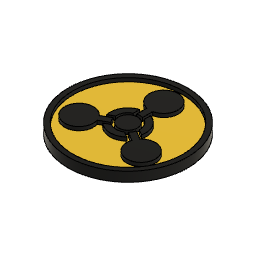
Chemical_symbol (Autodesk Fusion 360 design; units mm, degrees)
Autodesk Fusion 360 part; units mm, degrees
sketch "Sketch1" plane through (0, 0, 0) normal (0, 0, 1) x (1, 0, 0)
  circle A0 centre (0, 0) radius 25
  dimension "d1" = 50
  constraint coincident A0.centre origin
  measures "d1" diameter of A0
extrude "Extrude1" add sketch "Sketch1" along normal blind 2.5
sketch "Sketch2" plane through (0, 0, 2.5) normal (0, 0, 1) x (-1, 0, 0)
  circle A0 centre (0, 0) radius 25
  circle A1 centre (0, 0) radius 23
  circle A2 centre (0, 0) radius 21 construction
  circle A3 centre (0, 0) radius 4
  line L0 (0, 0) -> (0, -21) construction
  line L1 (0, 0) -> (-18.1865, 10.5) construction
  line L2 (18.1865, 10.5) -> (0, 0) construction
  line L3 (18.1865, 10.5) -> (0, -21) construction
  line L4 (-18.1865, 10.5) -> (0, -21) construction
  line L5 (-18.1865, 10.5) -> (18.1865, 10.5) construction
  circle A4 centre (0, 0) radius 5
  circle A5 centre (0, 0) radius 15 construction
  circle A6 centre (0, -15) radius 6
  circle A7 centre (-12.9904, 7.5) radius 6
  circle A8 centre (12.9904, 7.5) radius 6
  line L6 (8.5332, 3.4833) -> (3.9156, 0.8173)
  line L7 (7.2832, 5.6484) -> (2.6656, 2.9824)
  line L8 (8.5332, 3.4833) -> (7.2832, 5.6484) construction
  line L9 (3.9156, 0.8173) -> (2.6656, 2.9824) construction
  line L10 (-7.2832, 5.6484) -> (-2.6656, 2.9824)
  line L11 (-8.5332, 3.4833) -> (-3.9156, 0.8173)
  line L12 (-2.6656, 2.9824) -> (-3.9156, 0.8173) construction
  line L13 (-7.2832, 5.6484) -> (-8.5332, 3.4833) construction
  line L14 (-1.25, -9.1317) -> (-1.25, -3.7997)
  line L15 (1.25, -9.1317) -> (1.25, -3.7997)
  line L16 (-1.25, -3.7997) -> (1.25, -3.7997) construction
  line L17 (-1.25, -9.1317) -> (1.25, -9.1317) construction
  circle A9 centre (0, 0) radius 7.5
  line L18 (5.071, 5.5258) -> (2.7419, 4.1811)
  line L19 (7.321, 1.6287) -> (4.9919, 0.284)
  line L20 (-7.321, 1.6287) -> (-4.9919, 0.284)
  line L21 (-5.071, 5.5258) -> (-2.7419, 4.1811)
  line L22 (2.25, -7.1545) -> (2.25, -4.4651)
  line L23 (-2.25, -7.1545) -> (-2.25, -4.4651)
  dimension "d4" = -2
  dimension "d5" = -4
  dimension "d6" = 8
  dimension "d7" = 1
  dimension "d8" = -10
  dimension "d13" = 360
  dimension "d14" = 2.5
  dimension "d15" = 3.5
  dimension "d17" = 360
  dimension "d20" = 1
  constraint coincident A0.centre A1.centre
  constraint coincident A2 L0.end
  constraint vertical L0
  constraint coincident A2 L1.end
  constraint coincident A2 L2.start
  constraint equal L3 L4
  constraint equal L4 L5
  constraint coincident A5 A6.centre
  constraint coincident L0 A6.centre
  constraint coincident L1 A7.centre
  constraint coincident A5 A7.centre
  constraint coincident A5 A8.centre
  constraint coincident L2 A8.centre
  constraint coincident A8 L6.start
  constraint coincident A3 L6.end
  constraint coincident A8 L7.start
  constraint coincident A3 L7.end
  constraint parallel L6 L7
  constraint perpendicular L6 L8
  constraint perpendicular L7 L9
  constraint coincident A9 L18.start
  constraint coincident A4 L18.end
  constraint parallel L7 L18
  constraint symmetric L2 L18.start L19.start
  constraint symmetric L2 L18.end L19.end
  constraint tangent A2 A8
  constraint tangent A2 A7
  constraint tangent A2 A6
  measures "d6" diameter of A3
  measures "d14" distance of L6 L7
  measures "d20" distance of L7 L18
extrude "Extrude2" add sketch "Sketch2" along normal blind 1.5 contours A0 | A3 | A4 L6 L7 A9 | A4 L14 L15 A9 | A4 A9 L19 L22 | A8 L6 L7 A9 | A6 L14 L15 A9 | A4 L10 L11 A9 | A4 A9 L18 L21 | A8 | A4 A9 L20 L23 | A6 | A7 L10 L11 A9 | A7
